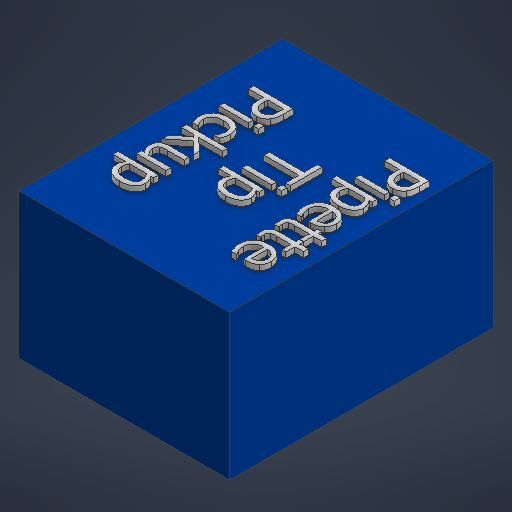
# Autodesk Inventor part: TipPickup
Saved by Autodesk Inventor 2025.1 (Build 291241000, 241)
## iProperties
Created: 2024-10-04
Part Number: TipPickup
Material: Generic
Document SubType Name: Modeling
Designer: jerem
Density: 1 g/cm^3
Appearance: Default
Author: jerem
Autodesk Inventor part; units mm, degrees
ref_plane "YZ Plane" through (0, 0, 0) normal (1, 0, 0) x (0, 1, 0)
ref_plane "XZ Plane" through (0, 0, 0) normal (0, 1, 0) x (-1, 0, 0)
ref_plane "XY Plane" through (0, 0, 0) normal (0, 0, 1) x (1, 0, 0)
sketch "Sketch1" plane through (0, 0, 0) normal (0, 1, 0) x (-1, 0, 0)
  line L0 (-40, -50) -> (40, -50)
  line L1 (40, -50) -> (40, 50)
  line L2 (40, 50) -> (-40, 50)
  line L3 (-40, 50) -> (-40, -50)
  line L4 (-40, -50) -> (40, 50) construction
  line L5 (40, -50) -> (-40, 50) construction
  point P0 (0, 0)
  dimension "d0" = 80
  dimension "d1" = 100
  constraints: 12 end point, 2 midpoint, 2 parallel, 1 horizontal, 1 perpendicular
  measures "d0" distance of L2.end L1.end
  measures "d1" distance of L1.end L0.end
extrude "Extrusion1" add sketch "Sketch1" along normal blind 55
sketch "Sketch2" plane through (0, 55, 0) normal (0, 1, 0) x (1, 0, 0)
  line L0 (26.4374, 11.3133) -> (26.4374, -13.2187) construction
  line L1 (26.4374, -13.2187) -> (-21.6739, -13.2187) construction
  line L2 (-21.6739, -13.2187) -> (-21.6739, 11.3133) construction
  line L3 (-21.6739, 11.3133) -> (26.4374, 11.3133) construction
  spline S0 degree 2 poles (32.0809, 19.5538) (31.1084, 19.5538) (29.358, 20.2467) (28.7502, 20.8666) knots 0 0 0 1 2 2 2
  spline S1 degree 2 poles (28.7502, 20.8666) (27.9844, 21.6445) (27.1943, 23.7475) (27.1943, 25.352) knots 0 0 0 1 2 2 2
  line L4 (27.1943, 25.352) -> (27.1943, 27.0416)
  line L5 (27.1943, 27.0416) -> (21.6028, 27.0416)
  line L6 (21.6028, 27.0416) -> (21.6028, 29.0351)
  line L7 (21.6028, 29.0351) -> (36.6028, 29.0351)
  line L8 (36.6028, 29.0351) -> (36.6028, 25.2669)
  spline S2 degree 2 poles (36.6028, 25.2669) (36.6028, 23.9298) (36.1652, 22.0578) (35.6668, 21.3407) knots 0 0 0 1 2 2 2
  spline S3 degree 2 poles (35.6668, 21.3407) (35.0955, 20.5019) (33.3329, 19.5538) (32.0809, 19.5538) knots 0 0 0 1 2 2 2
  spline S4 degree 2 poles (32.0201, 21.6324) (32.7981, 21.6324) (33.9407, 22.1672) (34.3054, 22.7142) knots 0 0 0 1 2 2 2
  spline S5 degree 2 poles (34.3054, 22.7142) (34.6214, 23.1883) (34.8767, 24.4525) (34.8767, 25.3885) knots 0 0 0 1 2 2 2
  line L9 (34.8767, 25.3885) -> (34.8767, 27.0416)
  line L10 (34.8767, 27.0416) -> (28.8961, 27.0416)
  line L11 (28.8961, 27.0416) -> (28.8961, 25.6802)
  spline S6 degree 2 poles (28.8961, 25.6802) (28.8961, 24.4646) (29.2851, 22.9695) (29.7956, 22.4833) knots 0 0 0 1 2 2 2
  spline S7 degree 2 poles (29.7956, 22.4833) (30.2454, 22.0335) (31.3029, 21.6324) (32.0201, 21.6324) knots 0 0 0 1 2 2 2
  line L12 (21.6028, 15.8706) -> (21.6028, 17.7669)
  line L13 (21.6028, 17.7669) -> (32.8588, 17.7669)
  line L14 (32.8588, 17.7669) -> (32.8588, 15.8706)
  line L15 (32.8588, 15.8706) -> (21.6028, 15.8706)
  line L16 (34.7308, 15.7369) -> (34.7308, 17.8885)
  line L17 (34.7308, 17.8885) -> (36.7, 17.8885)
  line L18 (36.7, 17.8885) -> (36.7, 15.7369)
  line L19 (36.7, 15.7369) -> (34.7308, 15.7369)
  spline S8 degree 2 poles (27.5347, 3.6543) (24.7146, 3.6543) (21.384, 6.3407) (21.384, 8.395) knots 0 0 0 1 2 2 2
  spline S9 degree 2 poles (21.384, 8.395) (21.384, 9.2337) (21.7729, 10.5222) (22.1741, 11.1907) knots 0 0 0 1 2 2 2
  line L20 (22.1741, 11.1907) -> (17.4577, 11.1907)
  line L21 (17.4577, 11.1907) -> (17.4577, 13.087)
  line L22 (17.4577, 13.087) -> (32.8588, 13.087)
  line L23 (32.8588, 13.087) -> (32.8588, 11.1907)
  line L24 (32.8588, 11.1907) -> (31.6797, 11.1907)
  spline S10 degree 2 poles (31.6797, 11.1907) (32.324, 10.4857) (33.1749, 8.7596) (33.1749, 7.7507) knots 0 0 0 1 2 2 2
  spline S11 degree 2 poles (33.1749, 7.7507) (33.1749, 5.818) (30.1117, 3.6543) (27.5347, 3.6543) knots 0 0 0 1 2 2 2
  spline S12 degree 2 poles (27.3159, 5.6113) (29.2486, 5.6113) (31.3759, 6.839) (31.3759, 8.2126) knots 0 0 0 1 2 2 2
  spline S13 degree 2 poles (31.3759, 8.2126) (31.3759, 9.0149) (30.6587, 10.5222) (30.0995, 11.1907) knots 0 0 0 1 2 2 2
  line L25 (30.0995, 11.1907) -> (23.7057, 11.1907)
  spline S14 degree 2 poles (23.7057, 11.1907) (23.3532, 10.4492) (23.0857, 9.3917) (23.0857, 8.711) knots 0 0 0 1 2 2 2
  spline S15 degree 2 poles (23.0857, 8.711) (23.0857, 7.2402) (25.2494, 5.6113) (27.3159, 5.6113) knots 0 0 0 1 2 2 2
  spline S16 degree 2 poles (21.3475, -3.2015) (21.3475, -0.5029) (24.3742, 2.463) (27.17, 2.463) knots 0 0 0 1 2 2 2
  spline S17 degree 2 poles (27.17, 2.463) (29.9172, 2.463) (33.1749, -0.4179) (33.1749, -2.7396) knots 0 0 0 1 2 2 2
  spline S18 degree 2 poles (33.1749, -2.7396) (33.1749, -3.785) (32.5671, -5.4016) (31.9229, -5.9973) knots 0 0 0 1 2 2 2
  spline S19 degree 2 poles (31.9229, -5.9973) (31.2786, -6.605) (29.4188, -7.2493) (28.0695, -7.2493) knots 0 0 0 1 2 2 2
  line L26 (28.0695, -7.2493) -> (27.0363, -7.2493)
  line L27 (27.0363, -7.2493) -> (27.0363, 0.5424)
  spline S20 degree 2 poles (27.0363, 0.5424) (25.0793, 0.5424) (23.0007, -1.4268) (23.0007, -3.1772) knots 0 0 0 1 2 2 2
  spline S21 degree 2 poles (23.0007, -3.1772) (23.0007, -3.7971) (23.2802, -5.0005) (23.499, -5.4867) knots 0 0 0 1 2 2 2
  spline S22 degree 2 poles (23.499, -5.4867) (23.7421, -5.9973) (24.1676, -6.7023) (24.3621, -6.9332) knots 0 0 0 1 2 2 2
  line L28 (24.3621, -6.9332) -> (24.3621, -7.0426)
  line L29 (24.3621, -7.0426) -> (22.2956, -7.0426)
  spline S23 degree 2 poles (22.2956, -7.0426) (22.1619, -6.7144) (21.7729, -5.7177) (21.6635, -5.3287) knots 0 0 0 1 2 2 2
  spline S24 degree 2 poles (21.6635, -5.3287) (21.5055, -4.7817) (21.3475, -3.8822) (21.3475, -3.2015) knots 0 0 0 1 2 2 2
  spline S25 degree 2 poles (28.4828, -5.4016) (29.2486, -5.3773) (30.3669, -5.0613) (30.7438, -4.7574) knots 0 0 0 1 2 2 2
  spline S26 degree 2 poles (30.7438, -4.7574) (31.1692, -4.4292) (31.619, -3.396) (31.619, -2.6302) knots 0 0 0 1 2 2 2
  spline S27 degree 2 poles (31.619, -2.6302) (31.619, -1.8765) (31.1692, -0.819) (30.7316, -0.3814) knots 0 0 0 1 2 2 2
  spline S28 degree 2 poles (30.7316, -0.3814) (30.2819, 0.0441) (29.2, 0.4817) (28.4828, 0.5424) knots 0 0 0 1 2 2 2
  line L30 (28.4828, 0.5424) -> (28.4828, -5.4016)
  spline S29 degree 2 poles (21.384, -12.5734) (21.384, -11.0297) (23.1465, -9.2914) (25.0549, -9.2914) knots 0 0 0 1 2 2 2
  line L31 (25.0549, -9.2914) -> (31.2908, -9.2914)
  line L32 (31.2908, -9.2914) -> (31.2908, -8.0151)
  line L33 (31.2908, -8.0151) -> (32.8588, -8.0151)
  line L34 (32.8588, -8.0151) -> (32.8588, -9.2914)
  line L35 (32.8588, -9.2914) -> (36.0922, -9.2914)
  line L36 (36.0922, -9.2914) -> (36.0922, -11.1877)
  line L37 (36.0922, -11.1877) -> (32.8588, -11.1877)
  line L38 (32.8588, -11.1877) -> (32.8588, -14.6764)
  line L39 (32.8588, -14.6764) -> (31.2908, -14.6764)
  line L40 (31.2908, -14.6764) -> (31.2908, -11.1877)
  line L41 (31.2908, -11.1877) -> (25.9301, -11.1877)
  spline S30 degree 2 poles (25.9301, -11.1877) (25.0793, -11.1877) (24.1433, -11.2485) (23.7421, -11.4551) knots 0 0 0 1 2 2 2
  spline S31 degree 2 poles (23.7421, -11.4551) (23.3896, -11.6253) (23.0371, -12.3911) (23.0371, -13.0475) knots 0 0 0 1 2 2 2
  spline S32 degree 2 poles (23.0371, -13.0475) (23.0371, -13.5094) (23.3167, -14.3725) (23.4018, -14.567) knots 0 0 0 1 2 2 2
  line L42 (23.4018, -14.567) -> (23.4018, -14.6764)
  line L43 (23.4018, -14.6764) -> (21.7, -14.6764)
  spline S33 degree 2 poles (21.7, -14.6764) (21.5541, -14.1415) (21.384, -13.0475) (21.384, -12.5734) knots 0 0 0 1 2 2 2
  spline S34 degree 2 poles (21.384, -19.4778) (21.384, -17.9341) (23.1465, -16.1958) (25.0549, -16.1958) knots 0 0 0 1 2 2 2
  line L44 (25.0549, -16.1958) -> (31.2908, -16.1958)
  line L45 (31.2908, -16.1958) -> (31.2908, -14.9195)
  line L46 (31.2908, -14.9195) -> (32.8588, -14.9195)
  line L47 (32.8588, -14.9195) -> (32.8588, -16.1958)
  line L48 (32.8588, -16.1958) -> (36.0922, -16.1958)
  line L49 (36.0922, -16.1958) -> (36.0922, -18.0921)
  line L50 (36.0922, -18.0921) -> (32.8588, -18.0921)
  line L51 (32.8588, -18.0921) -> (32.8588, -21.5807)
  line L52 (32.8588, -21.5807) -> (31.2908, -21.5807)
  line L53 (31.2908, -21.5807) -> (31.2908, -18.0921)
  line L54 (31.2908, -18.0921) -> (25.9301, -18.0921)
  spline S35 degree 2 poles (25.9301, -18.0921) (25.0793, -18.0921) (24.1433, -18.1529) (23.7421, -18.3595) knots 0 0 0 1 2 2 2
  spline S36 degree 2 poles (23.7421, -18.3595) (23.3896, -18.5297) (23.0371, -19.2955) (23.0371, -19.9519) knots 0 0 0 1 2 2 2
  spline S37 degree 2 poles (23.0371, -19.9519) (23.0371, -20.4138) (23.3167, -21.2768) (23.4018, -21.4713) knots 0 0 0 1 2 2 2
  line L55 (23.4018, -21.4713) -> (23.4018, -21.5807)
  line L56 (23.4018, -21.5807) -> (21.7, -21.5807)
  spline S38 degree 2 poles (21.7, -21.5807) (21.5541, -21.0459) (21.384, -19.9519) (21.384, -19.4778) knots 0 0 0 1 2 2 2
  spline S39 degree 2 poles (21.3475, -27.8652) (21.3475, -25.1666) (24.3742, -22.2007) (27.17, -22.2007) knots 0 0 0 1 2 2 2
  spline S40 degree 2 poles (27.17, -22.2007) (29.9172, -22.2007) (33.1749, -25.0815) (33.1749, -27.4033) knots 0 0 0 1 2 2 2
  spline S41 degree 2 poles (33.1749, -27.4033) (33.1749, -28.4486) (32.5671, -30.0653) (31.9229, -30.661) knots 0 0 0 1 2 2 2
  spline S42 degree 2 poles (31.9229, -30.661) (31.2786, -31.2687) (29.4188, -31.913) (28.0695, -31.913) knots 0 0 0 1 2 2 2
  line L57 (28.0695, -31.913) -> (27.0363, -31.913)
  line L58 (27.0363, -31.913) -> (27.0363, -24.1213)
  spline S43 degree 2 poles (27.0363, -24.1213) (25.0793, -24.1213) (23.0007, -26.0905) (23.0007, -27.8409) knots 0 0 0 1 2 2 2
  spline S44 degree 2 poles (23.0007, -27.8409) (23.0007, -28.4608) (23.2802, -29.6642) (23.499, -30.1504) knots 0 0 0 1 2 2 2
  spline S45 degree 2 poles (23.499, -30.1504) (23.7421, -30.661) (24.1676, -31.366) (24.3621, -31.5969) knots 0 0 0 1 2 2 2
  line L59 (24.3621, -31.5969) -> (24.3621, -31.7063)
  line L60 (24.3621, -31.7063) -> (22.2956, -31.7063)
  spline S46 degree 2 poles (22.2956, -31.7063) (22.1619, -31.3781) (21.7729, -30.3814) (21.6635, -29.9924) knots 0 0 0 1 2 2 2
  spline S47 degree 2 poles (21.6635, -29.9924) (21.5055, -29.4454) (21.3475, -28.5459) (21.3475, -27.8652) knots 0 0 0 1 2 2 2
  spline S48 degree 2 poles (28.4828, -30.0653) (29.2486, -30.041) (30.3669, -29.725) (30.7438, -29.4211) knots 0 0 0 1 2 2 2
  spline S49 degree 2 poles (30.7438, -29.4211) (31.1692, -29.0929) (31.619, -28.0597) (31.619, -27.2939) knots 0 0 0 1 2 2 2
  spline S50 degree 2 poles (31.619, -27.2939) (31.619, -26.5402) (31.1692, -25.4827) (30.7316, -25.0451) knots 0 0 0 1 2 2 2
  spline S51 degree 2 poles (30.7316, -25.0451) (30.2819, -24.6196) (29.2, -24.182) (28.4828, -24.1213) knots 0 0 0 1 2 2 2
  line L61 (28.4828, -24.1213) -> (28.4828, -30.0653)
  line L62 (-3.0943, 8.1093) -> (10.1309, 8.1093)
  line L63 (10.1309, 8.1093) -> (10.1309, 13.1417)
  line L64 (10.1309, 13.1417) -> (11.9057, 13.1417)
  line L65 (11.9057, 13.1417) -> (11.9057, 1.0834)
  line L66 (11.9057, 1.0834) -> (10.1309, 1.0834)
  line L67 (10.1309, 1.0834) -> (10.1309, 6.1158)
  line L68 (10.1309, 6.1158) -> (-3.0943, 6.1158)
  line L69 (-3.0943, 6.1158) -> (-3.0943, 8.1093)
  line L70 (-3.0943, -2.223) -> (-3.0943, -0.3267)
  line L71 (-3.0943, -0.3267) -> (8.1617, -0.3267)
  line L72 (8.1617, -0.3267) -> (8.1617, -2.223)
  line L73 (8.1617, -2.223) -> (-3.0943, -2.223)
  line L74 (10.0337, -2.3567) -> (10.0337, -0.2051)
  line L75 (10.0337, -0.2051) -> (12.0029, -0.2051)
  line L76 (12.0029, -0.2051) -> (12.0029, -2.3567)
  line L77 (12.0029, -2.3567) -> (10.0337, -2.3567)
  spline S52 degree 2 poles (2.8376, -14.4393) (0.0175, -14.4393) (-3.3131, -11.7529) (-3.3131, -9.6986) knots 0 0 0 1 2 2 2
  spline S53 degree 2 poles (-3.3131, -9.6986) (-3.3131, -8.8599) (-2.9242, -7.5714) (-2.523, -6.9029) knots 0 0 0 1 2 2 2
  line L78 (-2.523, -6.9029) -> (-7.2394, -6.9029)
  line L79 (-7.2394, -6.9029) -> (-7.2394, -5.0066)
  line L80 (-7.2394, -5.0066) -> (8.1617, -5.0066)
  line L81 (8.1617, -5.0066) -> (8.1617, -6.9029)
  line L82 (8.1617, -6.9029) -> (6.9826, -6.9029)
  spline S54 degree 2 poles (6.9826, -6.9029) (7.6269, -7.6079) (8.4778, -9.334) (8.4778, -10.3429) knots 0 0 0 1 2 2 2
  spline S55 degree 2 poles (8.4778, -10.3429) (8.4778, -12.2756) (5.4146, -14.4393) (2.8376, -14.4393) knots 0 0 0 1 2 2 2
  spline S56 degree 2 poles (2.6188, -12.4823) (4.5515, -12.4823) (6.6787, -11.2546) (6.6787, -9.881) knots 0 0 0 1 2 2 2
  spline S57 degree 2 poles (6.6787, -9.881) (6.6787, -9.0787) (5.9616, -7.5714) (5.4024, -6.9029) knots 0 0 0 1 2 2 2
  line L83 (5.4024, -6.9029) -> (-0.9914, -6.9029)
  spline S58 degree 2 poles (-0.9914, -6.9029) (-1.3439, -7.6444) (-1.6114, -8.7019) (-1.6114, -9.3826) knots 0 0 0 1 2 2 2
  spline S59 degree 2 poles (-1.6114, -9.3826) (-1.6114, -10.8534) (0.5523, -12.4823) (2.6188, -12.4823) knots 0 0 0 1 2 2 2
  spline S60 degree 2 poles (-17.3133, 17.4387) (-18.2858, 17.4387) (-20.0362, 18.1316) (-20.644, 18.7515) knots 0 0 0 1 2 2 2
  spline S61 degree 2 poles (-20.644, 18.7515) (-21.4098, 19.5295) (-22.1999, 21.6324) (-22.1999, 23.2369) knots 0 0 0 1 2 2 2
  line L84 (-22.1999, 23.2369) -> (-22.1999, 24.9266)
  line L85 (-22.1999, 24.9266) -> (-27.7915, 24.9266)
  line L86 (-27.7915, 24.9266) -> (-27.7915, 26.9201)
  line L87 (-27.7915, 26.9201) -> (-12.7915, 26.9201)
  line L88 (-12.7915, 26.9201) -> (-12.7915, 23.1518)
  spline S62 degree 2 poles (-12.7915, 23.1518) (-12.7915, 21.8147) (-13.2291, 19.9428) (-13.7274, 19.2256) knots 0 0 0 1 2 2 2
  spline S63 degree 2 poles (-13.7274, 19.2256) (-14.2987, 18.3868) (-16.0613, 17.4387) (-17.3133, 17.4387) knots 0 0 0 1 2 2 2
  spline S64 degree 2 poles (-17.3741, 19.5173) (-16.5962, 19.5173) (-15.4535, 20.0522) (-15.0889, 20.5992) knots 0 0 0 1 2 2 2
  spline S65 degree 2 poles (-15.0889, 20.5992) (-14.7728, 21.0732) (-14.5175, 22.3374) (-14.5175, 23.2734) knots 0 0 0 1 2 2 2
  line L89 (-14.5175, 23.2734) -> (-14.5175, 24.9266)
  line L90 (-14.5175, 24.9266) -> (-20.4981, 24.9266)
  line L91 (-20.4981, 24.9266) -> (-20.4981, 23.5651)
  spline S66 degree 2 poles (-20.4981, 23.5651) (-20.4981, 22.3496) (-20.1091, 20.8544) (-19.5986, 20.3682) knots 0 0 0 1 2 2 2
  spline S67 degree 2 poles (-19.5986, 20.3682) (-19.1488, 19.9185) (-18.0913, 19.5173) (-17.3741, 19.5173) knots 0 0 0 1 2 2 2
  line L92 (-27.7915, 13.7556) -> (-27.7915, 15.6518)
  line L93 (-27.7915, 15.6518) -> (-16.5354, 15.6518)
  line L94 (-16.5354, 15.6518) -> (-16.5354, 13.7556)
  line L95 (-16.5354, 13.7556) -> (-27.7915, 13.7556)
  line L96 (-14.6634, 13.6219) -> (-14.6634, 15.7734)
  line L97 (-14.6634, 15.7734) -> (-12.6942, 15.7734)
  line L98 (-12.6942, 15.7734) -> (-12.6942, 13.6219)
  line L99 (-12.6942, 13.6219) -> (-14.6634, 13.6219)
  spline S68 degree 2 poles (-28.0467, 6.4987) (-28.0467, 7.6656) (-27.3295, 9.5984) (-26.6002, 10.2912) knots 0 0 0 1 2 2 2
  spline S69 degree 2 poles (-26.6002, 10.2912) (-25.883, 10.9841) (-23.6707, 11.7499) (-22.1877, 11.7499) knots 0 0 0 1 2 2 2
  spline S70 degree 2 poles (-22.1877, 11.7499) (-20.7047, 11.7499) (-18.541, 10.9598) (-17.8117, 10.2912) knots 0 0 0 1 2 2 2
  spline S71 degree 2 poles (-17.8117, 10.2912) (-17.0702, 9.6227) (-16.2801, 7.6413) (-16.2801, 6.4987) knots 0 0 0 1 2 2 2
  spline S72 degree 2 poles (-16.2801, 6.4987) (-16.2801, 5.5749) (-16.8028, 3.8488) (-17.1432, 3.1802) knots 0 0 0 1 2 2 2
  line L100 (-17.1432, 3.1802) -> (-19.2704, 3.1802)
  line L101 (-19.2704, 3.1802) -> (-19.2704, 3.2896)
  spline S73 degree 2 poles (-19.2704, 3.2896) (-19.1002, 3.4962) (-18.6626, 4.1283) (-18.4316, 4.5781) knots 0 0 0 1 2 2 2
  spline S74 degree 2 poles (-18.4316, 4.5781) (-18.2372, 4.9792) (-17.9333, 6.0489) (-17.9333, 6.5351) knots 0 0 0 1 2 2 2
  spline S75 degree 2 poles (-17.9333, 6.5351) (-17.9333, 8.006) (-20.1577, 9.7928) (-22.1877, 9.7928) knots 0 0 0 1 2 2 2
  spline S76 degree 2 poles (-22.1877, 9.7928) (-24.1691, 9.7928) (-26.3936, 8.0668) (-26.3936, 6.5351) knots 0 0 0 1 2 2 2
  spline S77 degree 2 poles (-26.3936, 6.5351) (-26.3936, 5.6113) (-25.6278, 3.9338) (-25.0321, 3.2896) knots 0 0 0 1 2 2 2
  line L102 (-25.0321, 3.2896) -> (-25.0321, 3.1802)
  line L103 (-25.0321, 3.1802) -> (-27.1594, 3.1802)
  spline S78 degree 2 poles (-27.1594, 3.1802) (-27.2931, 3.4598) (-27.6699, 4.3107) (-27.755, 4.651) knots 0 0 0 1 2 2 2
  spline S79 degree 2 poles (-27.755, 4.651) (-27.9009, 5.1373) (-28.0467, 5.9031) (-28.0467, 6.4987) knots 0 0 0 1 2 2 2
  line L104 (-27.7915, -7.8692) -> (-27.7915, -5.3773)
  line L105 (-27.7915, -5.3773) -> (-22.3579, -1.1958)
  line L106 (-22.3579, -1.1958) -> (-23.0872, -0.4422)
  line L107 (-23.0872, -0.4422) -> (-27.7915, -0.4422)
  line L108 (-27.7915, -0.4422) -> (-27.7915, 1.4541)
  line L109 (-27.7915, 1.4541) -> (-12.1229, 1.4541)
  line L110 (-12.1229, 1.4541) -> (-12.1229, -0.4422)
  line L111 (-12.1229, -0.4422) -> (-21.2882, -0.4422)
  line L112 (-21.2882, -0.4422) -> (-16.5354, -4.8911)
  line L113 (-16.5354, -4.8911) -> (-16.5354, -7.2493)
  line L114 (-16.5354, -7.2493) -> (-21.2396, -2.6302)
  line L115 (-21.2396, -2.6302) -> (-27.7915, -7.8692)
  line L116 (-27.7915, -17.5694) -> (-27.7915, -15.6731)
  line L117 (-27.7915, -15.6731) -> (-26.5516, -15.6731)
  spline S80 degree 2 poles (-26.5516, -15.6731) (-27.3174, -14.7979) (-28.1075, -13.2298) (-28.1075, -12.2574) knots 0 0 0 1 2 2 2
  spline S81 degree 2 poles (-28.1075, -12.2574) (-28.1075, -11.5281) (-27.6213, -10.2274) (-27.0986, -9.7533) knots 0 0 0 1 2 2 2
  spline S82 degree 2 poles (-27.0986, -9.7533) (-26.5759, -9.2671) (-24.9835, -8.7323) (-23.8409, -8.7323) knots 0 0 0 1 2 2 2
  line L118 (-23.8409, -8.7323) -> (-16.5354, -8.7323)
  line L119 (-16.5354, -8.7323) -> (-16.5354, -10.6285)
  line L120 (-16.5354, -10.6285) -> (-22.9535, -10.6285)
  spline S83 degree 2 poles (-22.9535, -10.6285) (-23.853, -10.6285) (-25.0321, -10.7623) (-25.4697, -10.9932) knots 0 0 0 1 2 2 2
  spline S84 degree 2 poles (-25.4697, -10.9932) (-25.9073, -11.2242) (-26.3085, -12.0143) (-26.3085, -12.7558) knots 0 0 0 1 2 2 2
  spline S85 degree 2 poles (-26.3085, -12.7558) (-26.3085, -13.4486) (-25.5184, -15.0167) (-24.947, -15.6731) knots 0 0 0 1 2 2 2
  line L121 (-24.947, -15.6731) -> (-16.5354, -15.6731)
  line L122 (-16.5354, -15.6731) -> (-16.5354, -17.5694)
  line L123 (-16.5354, -17.5694) -> (-27.7915, -17.5694)
  spline S86 degree 2 poles (-21.8595, -29.7493) (-24.6796, -29.7493) (-28.0103, -27.0629) (-28.0103, -25.0086) knots 0 0 0 1 2 2 2
  spline S87 degree 2 poles (-28.0103, -25.0086) (-28.0103, -24.1699) (-27.6213, -22.8814) (-27.2201, -22.2128) knots 0 0 0 1 2 2 2
  line L124 (-27.2201, -22.2128) -> (-31.9365, -22.2128)
  line L125 (-31.9365, -22.2128) -> (-31.9365, -20.3166)
  line L126 (-31.9365, -20.3166) -> (-16.5354, -20.3166)
  line L127 (-16.5354, -20.3166) -> (-16.5354, -22.2128)
  line L128 (-16.5354, -22.2128) -> (-17.7145, -22.2128)
  spline S88 degree 2 poles (-17.7145, -22.2128) (-17.0702, -22.9179) (-16.2193, -24.6439) (-16.2193, -25.6529) knots 0 0 0 1 2 2 2
  spline S89 degree 2 poles (-16.2193, -25.6529) (-16.2193, -27.5856) (-19.2825, -29.7493) (-21.8595, -29.7493) knots 0 0 0 1 2 2 2
  spline S90 degree 2 poles (-22.0783, -27.7922) (-20.1456, -27.7922) (-18.0184, -26.5645) (-18.0184, -25.1909) knots 0 0 0 1 2 2 2
  spline S91 degree 2 poles (-18.0184, -25.1909) (-18.0184, -24.3887) (-18.7355, -22.8814) (-19.2947, -22.2128) knots 0 0 0 1 2 2 2
  line L129 (-19.2947, -22.2128) -> (-25.6885, -22.2128)
  spline S92 degree 2 poles (-25.6885, -22.2128) (-26.041, -22.9543) (-26.3085, -24.0119) (-26.3085, -24.6926) knots 0 0 0 1 2 2 2
  spline S93 degree 2 poles (-26.3085, -24.6926) (-26.3085, -26.1634) (-24.1448, -27.7922) (-22.0783, -27.7922) knots 0 0 0 1 2 2 2
  point P0 (0, 0)
  constraints: 2 other
extrude "Extrusion2" add sketch "Sketch2" along normal blind 2
body "Solid1"
